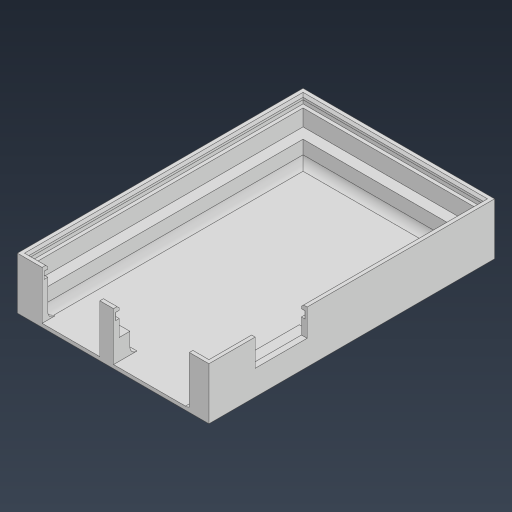
# Autodesk Inventor part: case
Saved by Autodesk Inventor 2023 (Build 270158000, 158)
## iProperties
Created: 2025-06-15
Part Number: case
Material: Generic
Document SubType Name: Modeling
Designer: szymo
Density: 1 g/cm^3
Appearance: Default
Author: szymo
Autodesk Inventor part; units mm, degrees
ref_plane "YZ Plane" through (0, 0, 0) normal (1, 0, 0) x (0, 1, 0)
ref_plane "Work Plane1" through (-26.0554, 5.5841, 57.3172) normal (0, -1, 0) x (1, 0, 0)
sketch "Sketch1" plane through (-26.0554, 5.5841, 57.3172) normal (0, -1, 0) x (1, 0, 0)
  arc A0 (-6.2529, -16.6318) -> (-5.7152, -17.8896) centre (-4.5084, -16.63) ccw projected
  line L0 (-6.2529, -16.6318) -> (-8.9554, -15.4715) projected
  arc A1 (-8.9554, -15.4715) -> (-9.6085, -15.4715) centre (-9.2819, -16.2321) ccw projected
  line L1 (-9.6085, -15.4715) -> (-11.5974, -15.1528) projected
  arc A2 (-11.5974, -15.1528) -> (-12.113, -13.8772) centre (-12.9119, -14.9421) ccw projected
  line L2 (-12.113, -13.8772) -> (-12.113, -11.7599) projected
  line L3 (-12.113, -11.7599) -> (-10.8096, -8.0503) projected
  line L4 (-10.8096, -8.0503) -> (-0.9192, -8.5103) projected
  arc A3 (-0.3314, -8.8426) -> (-0.9192, -8.5103) centre (-0.954, -9.258) ccw projected
  line L5 (-0.3314, -8.8426) -> (2.5309, -17.8896) projected
  arc A4 (2.5309, -18.6308) -> (2.5309, -17.8896) centre (1.3597, -18.2602) ccw projected
  line L6 (2.5309, -18.6308) -> (1.3597, -25.9399) projected
  line L7 (1.3597, -25.9399) -> (-2.6315, -30.1057) projected
  arc A5 (-3.5771, -30.3612) -> (-2.6315, -30.1057) centre (-3.3161, -29.4497) ccw projected
  line L8 (-3.5771, -30.3612) -> (-8.4584, -28.2656) projected
  arc A6 (-9.8385, -26.6044) -> (-8.4584, -28.2656) centre (-7.5216, -26.0835) ccw projected
  line L9 (-9.8385, -26.6044) -> (-9.8385, -22.4387) projected
  arc A7 (-9.6085, -21.9531) -> (-9.8385, -22.4387) centre (-9.2109, -22.4387) ccw projected
  line L10 (-9.6085, -21.9531) -> (-5.7152, -17.8896) projected
  line L11 (7.08, -38.1436) -> (-17.82, -38.1436) projected
  line L12 (7.08, 0) -> (7.08, -38.1436) projected
  line L13 (-17.12, 0) -> (7.08, 0) projected
  line L14 (-17.82, -38.1436) -> (-17.12, 0) projected
  line L15 (-15.12, 0) -> (-15.12, -2.1) projected
  line L16 (4.83, 0) -> (4.83, -2.3) projected
  line L17 (-7.5, -2.1) -> (-7.5, 0) projected
  line L18 (-5.08, 0) -> (-5.08, -2.1) projected
  line L19 (8.08, -39.1436) -> (-18.8385, -39.1436)
  line L20 (-18.8385, -39.1436) -> (-18.1018, 1)
  line L21 (-18.1018, 1) -> (8.08, 1)
  line L22 (8.08, 1) -> (8.08, -39.1436)
  line L23 (-18.8385, -39.1436) -> (-18.8385, 1)
  line L24 (-18.8385, 1) -> (-18.1018, 1)
  point P0 (26.0554, -57.3172)
  dimension "d2" = 1
  constraints: 12 end point, 1 parallel, 1 perpendicular, 3 other
  measures "d2" distance between parallel lines of L12 L22
extrude "Extrusion1" add sketch "Sketch1" along normal blind 0.5 contours L0 A1 L1 A2 L2 L3 L4 A3 L5 A4 L6 L7 A5 L8 A6 L9 A7 L10 A0 | L11 L14 L13 L12 | L19 L20 L21 L22 | L23 L24 L20
sketch "Sketch2" plane through (-26.0554, 5.5841, 57.3172) normal (0, 1, 0) x (1, 0, 0)
  line L0 (5.08, 0) -> (5.08, 2.1)
  line L1 (5.08, 2.1) -> (5.08, 0)
  line L2 (-5.08, 0) -> (-5.08, 2.1)
  line L3 (-7.5, 2.1) -> (-7.5, 0)
  line L4 (-15.12, 0) -> (-15.12, 2.1)
  line L5 (4.83, 2.3) -> (2.79, 2.3)
  line L6 (8.08, 39.1436) -> (8.08, -1)
  line L7 (-18.8385, 39.1436) -> (8.08, 39.1436)
  line L8 (5.08, 2.1) -> (5.08, 2.3)
  line L9 (5.08, 2.3) -> (4.83, 2.3)
  line L10 (2.79, 2.3) -> (-5.08, 2.3)
  line L11 (-5.08, 2.3) -> (-5.08, 2.0628)
  line L12 (-7.5, 2.1) -> (-7.5, 2.3)
  line L13 (-7.5, 2.3) -> (-15.12, 2.3)
  line L14 (-15.12, 2.3) -> (-15.12, 2.0628)
  line L15 (-7.5, 0) -> (-15.12, 0)
  line L16 (-5.08, 0) -> (5.08, 0)
  line L17 (8.08, -1) -> (-17.1109, -1)
  line L18 (-7.25, 2.55) -> (-15.37, 2.55)
  line L19 (-15.37, 2.55) -> (-15.37, -1)
  line L20 (-15.37, -1) -> (-7.25, -1)
  line L21 (-7.25, -1) -> (-7.25, 2.55)
  line L22 (-5.33, -1) -> (5.33, -1)
  line L23 (5.33, -1) -> (5.33, 2.55)
  line L24 (5.33, 2.55) -> (-5.33, 2.55)
  line L25 (-5.33, 2.55) -> (-5.33, -1)
  line L26 (8.08, -1) -> (-18.8385, -1)
  line L27 (-18.8385, -1) -> (-18.8385, 39.1436)
  line L28 (7.28, -0.2) -> (7.28, 38.3436)
  line L29 (7.28, 38.3436) -> (-18.0385, 38.3436)
  line L30 (-18.0385, 38.3436) -> (-18.0385, -0.2)
  line L31 (-18.0385, -0.2) -> (7.28, -0.2)
  point P0 (26.0554, 57.3172)
  point P1 (-5.33, -0.2)
  point P2 (-7.25, -0.2)
  point P3 (-7.25, -1)
  point P4 (-17.6109, -0.5)
  point P5 (-15.37, -0.2)
  point P6 (5.33, -0.2)
  point P7 (5.33, -1)
  point P8 (-17.1109, -1)
extrude "Extrusion2" add sketch "Sketch2" along normal blind 5.2 contours L6 L17 L23 L31 L28 L29 L30 L19 L26 L27 L7 | L17 L21 L31 L25
sketch "Sketch3" plane through (-17.9754, 5.0841, 58.3172) normal (1, 0, 0) x (0, 0, -1)
  line L0 (6.5, 4) -> (13.3, 4)
  line L1 (6.5, 7.65) -> (13.8, 7.65)
  line L2 (13.8, 7.65) -> (13.8, 3.5)
  line L3 (13.8, 3.5) -> (6.5, 3.5)
  line L4 (6.5, 3.5) -> (6.5, 7.65)
  line L5 (1, 3.4) -> (39.1436, 3.4) projected
  line L6 (39.1436, 3.4) -> (39.1436, 4) projected
  line L7 (13.3, 4) -> (39.1436, 4) projected
  line L8 (13.3, 4) -> (13.3, 7.15) projected
  line L9 (7, 7.15) -> (13.3, 7.15) projected
  line L10 (7, 4) -> (7, 7.15) projected
  line L11 (1, 4) -> (7, 4) projected
  line L12 (1, 3.4) -> (1, 4) projected
  point P0 (58.3172, -5.0841)
  dimension "d14" = 0.5
  dimension "d41" = 0.5
  dimension "d42" = 0.5
  dimension "d43" = 0.5
  constraints: 8 end point, 2 horizontal, 1 parallel, 1 vertical, 3 other
  measures "d14" distance between parallel lines of L3 L0
  measures "d41" distance between parallel lines of L4 L10
  measures "d42" distance between parallel lines of L9 L1
extrude "Extrusion3" cut sketch "Sketch3" against normal blind 5.2 contours L4 L1 L2 L7 L8 L9 L10 L0 | L0 L7 L2 L3 L4 | L10 L9 L8 L0
sketch "Sketch4" plane through (-26.0554, 10.7841, 57.3172) normal (0, 1, 0) x (1, 0, 0)
  line L0 (8.08, 5.5) -> (7.28, 5.5) projected
  line L1 (7.28, 5.5) -> (7.28, -0.2) projected
  line L2 (7.28, -0.2) -> (5.33, -0.2) projected
  line L3 (5.33, -0.2) -> (5.33, -1) projected
  line L4 (5.33, -1) -> (8.08, -1) projected
  line L5 (8.08, -1) -> (8.08, 5.5) projected
  line L6 (7.28, 12.8) -> (8.08, 12.8) projected
  line L7 (8.08, 12.8) -> (8.08, 39.1436) projected
  line L8 (8.08, 39.1436) -> (-18.8385, 39.1436) projected
  line L9 (-18.8385, 39.1436) -> (-18.8385, -1) projected
  line L10 (-18.8385, -1) -> (-15.37, -1) projected
  line L11 (-15.37, -1) -> (-15.37, -0.2) projected
  line L12 (-15.37, -0.2) -> (-18.0385, -0.2) projected
  line L13 (-18.0385, -0.2) -> (-18.0385, 38.3436) projected
  line L14 (-18.0385, 38.3436) -> (7.28, 38.3436) projected
  line L15 (7.28, 38.3436) -> (7.28, 12.8) projected
  line L16 (-7.25, -0.2) -> (-7.25, -1) projected
  line L17 (-7.25, -1) -> (-5.33, -1) projected
  line L18 (-5.33, -1) -> (-5.33, -0.2) projected
  line L19 (-5.33, -0.2) -> (-7.25, -0.2) projected
  line L20 (-15.37, -0.2) -> (-15.37, -1) projected
  line L21 (-15.37, -0.7) -> (-18.5385, -0.7)
  line L22 (-18.5385, -0.7) -> (-18.5385, 38.8436)
  line L23 (-18.5385, 38.8436) -> (7.78, 38.8436)
  line L24 (7.78, 38.8436) -> (7.78, 12.8)
  line L25 (7.78, 5.5) -> (7.78, -0.7)
  line L26 (7.78, -0.7) -> (5.33, -0.7)
  line L27 (-7.25, -0.7) -> (-5.33, -0.7)
  point P0 (8.08, 25.9718)
  point P1 (-15.37, -0.7)
  dimension "d44" = 0.3
  dimension "d45" = 0.3
  dimension "d46" = 0.3
  dimension "d47" = 0.3
  dimension "d48" = 0.3
  dimension "d49" = 0.3
  constraints: 14 end point, 7 perpendicular, 7 point on line, 1 horizontal, 1 midpoint, 1 parallel
  measures "d44" distance between parallel lines of L17 L27
  measures "d45" distance between parallel lines of L10 L21
  measures "d46" distance between parallel lines of L9 L22
  measures "d47" distance between parallel lines of L8 L23
  measures "d48" distance from line of point (8.08, 25.972) L24
  measures "d49" distance between parallel lines of L4 L26
extrude "Extrusion4" add sketch "Sketch4" along normal blind 1 contours L5 L4 L3 L26 L25 L0 | L24 L23 L22 L21 L11 L10 L9 L8 L7 L6 | L27 L18 L17 L16
sketch "Sketch5" plane through (-26.0554, 11.7841, 57.3172) normal (0, 1, 0) x (1, 0, 0)
  line L0 (-15.37, -1) -> (-15.37, -0.2) projected
  line L1 (8.08, 12.8) -> (8.08, 39.1436) projected
  line L2 (8.08, 39.1436) -> (-18.8385, 39.1436) projected
  line L3 (-18.8385, 39.1436) -> (-18.8385, -1) projected
  line L4 (-18.8385, -1) -> (-15.37, -1) projected
  line L5 (7.58, 5.5) -> (7.38, 5.5) projected
  line L6 (7.38, 5.5) -> (7.38, -0.3) projected
  line L7 (7.38, -0.3) -> (5.33, -0.3) projected
  line L8 (5.33, -0.3) -> (5.33, -0.5) projected
  line L9 (5.33, -0.5) -> (7.58, -0.5) projected
  line L10 (7.58, -0.5) -> (7.58, 5.5) projected
  line L11 (-7.25, -0.2) -> (-7.25, -1) projected
  line L12 (-7.25, -1) -> (-5.33, -1) projected
  line L13 (-15.37, -1) -> (-15.37, -0.2) projected
  line L14 (-15.37, -0.2) -> (-18.0385, -0.2) projected
  line L15 (-18.0385, -0.2) -> (-18.0385, 38.3436) projected
  line L16 (-18.0385, 38.3436) -> (7.28, 38.3436) projected
  line L17 (7.28, 38.3436) -> (7.28, 12.8) projected
  line L18 (-5.33, -0.2) -> (-7.25, -0.2) projected
  line L19 (-7.25, -0.2) -> (-7.25, -1) projected
  line L20 (7.28, 5.5) -> (7.28, -0.2) projected
  line L21 (7.28, -0.2) -> (5.33, -0.2) projected
  line L22 (-7.25, -0.2) -> (-7.25, -1) projected
  line L23 (-15.37, -1) -> (-15.37, -0.2) projected
  line L24 (-15.37, -0.2) -> (-18.0385, -0.2) projected
  line L25 (-18.0385, -0.2) -> (-18.0385, 38.3436) projected
  line L26 (-18.0385, 38.3436) -> (7.28, 38.3436) projected
  line L27 (-15.37, -1) -> (-15.37, -0.2) projected
  line L28 (-15.37, -0.2) -> (-18.0385, -0.2) projected
  line L29 (-18.0385, -0.2) -> (-18.0385, 38.3436) projected
  line L30 (-18.0385, 38.3436) -> (7.28, 38.3436) projected
  line L31 (7.28, 38.3436) -> (7.28, 12.8) projected
  line L32 (-7.25, -0.2) -> (-7.25, -1) projected
  line L33 (7.28, -0.2) -> (5.33, -0.2) projected
  line L34 (7.28, 12.8) -> (8.08, 12.8) projected
  line L35 (8.08, 12.8) -> (8.08, 39.1436) projected
  line L36 (8.08, 39.1436) -> (-18.8385, 39.1436) projected
  line L37 (-18.8385, 39.1436) -> (-18.8385, -1) projected
  line L38 (-18.8385, -1) -> (-15.37, -1) projected
  line L39 (8.08, -1) -> (8.08, 5.5) projected
  line L40 (8.08, 5.5) -> (7.28, 5.5) projected
  line L41 (7.28, 38.3436) -> (7.28, 12.8) projected
  line L42 (7.28, 12.8) -> (8.08, 12.8) projected
  line L43 (8.08, 12.8) -> (8.08, 39.1436) projected
  line L44 (8.08, 39.1436) -> (-18.8385, 39.1436) projected
  line L45 (-18.8385, 39.1436) -> (-18.8385, -1) projected
  line L46 (-18.8385, -1) -> (-15.37, -1) projected
  line L47 (8.08, -1) -> (8.08, 5.5) projected
  line L48 (8.08, 5.5) -> (7.28, 5.5) projected
  line L49 (7.28, 5.5) -> (7.28, -0.2) projected
  line L50 (7.28, 12.8) -> (8.08, 12.8) projected
  line L51 (8.08, 12.8) -> (8.08, 39.1436) projected
  line L52 (8.08, 39.1436) -> (-18.8385, 39.1436) projected
  line L53 (-18.8385, 39.1436) -> (-18.8385, -1) projected
  line L54 (-18.8385, -1) -> (-15.37, -1) projected
  line L55 (8.08, -1) -> (8.08, 5.5) projected
  line L56 (8.08, 5.5) -> (7.28, 5.5) projected
  line L57 (7.28, 5.5) -> (7.28, -0.2) projected
  line L58 (8.08, -1) -> (8.08, 5.5) projected
  line L59 (8.08, 5.5) -> (7.28, 5.5) projected
  line L60 (7.28, 5.5) -> (7.28, -0.2) projected
  line L61 (-5.33, -0.2) -> (-7.25, -0.2) projected
  line L62 (-7.25, -1) -> (-5.33, -1) projected
  line L63 (-5.33, -1) -> (-5.33, -0.2) projected
  line L64 (-5.33, -0.2) -> (-7.25, -0.2) projected
  line L65 (5.33, -0.2) -> (5.33, -1) projected
  line L66 (5.33, -1) -> (8.08, -1) projected
  line L67 (-7.25, -1) -> (-5.33, -1) projected
  line L68 (-5.33, -1) -> (-5.33, -0.2) projected
  line L69 (7.28, -0.2) -> (5.33, -0.2) projected
  line L70 (5.33, -0.2) -> (5.33, -1) projected
  line L71 (5.33, -1) -> (8.08, -1) projected
  line L72 (-7.25, -1) -> (-5.33, -1) projected
  line L73 (-5.33, -1) -> (-5.33, -0.2) projected
  line L74 (-5.33, -0.2) -> (-7.25, -0.2) projected
  line L75 (5.33, -0.2) -> (5.33, -1) projected
  line L76 (5.33, -1) -> (8.08, -1) projected
  line L77 (-5.33, -1) -> (-5.33, -0.2) projected
  line L78 (7.28, -0.2) -> (5.33, -0.2) projected
  line L79 (5.33, -0.2) -> (5.33, -1) projected
  line L80 (5.33, -1) -> (8.08, -1) projected
  line L81 (-15.37, -0.2) -> (-18.0385, -0.2) projected
  line L82 (-18.0385, -0.2) -> (-18.0385, 38.3436) projected
  line L83 (-18.0385, 38.3436) -> (7.28, 38.3436) projected
  line L84 (7.28, 38.3436) -> (7.28, 12.8) projected
  line L85 (7.28, 12.8) -> (8.08, 12.8) projected
  point P0 (26.0554, 57.3172)
extrude "Extrusion5" add sketch "Sketch5" along normal blind 0.6
chamfer "Chamfer1" distance 0.3 angle 45 7 edges at (-42.7597, 12.3841, 57.5172) (-44.0939, 12.3841, 38.2454) (-31.4347, 12.3841, 18.9736) (-18.7754, 12.3841, 31.7454) (-32.3454, 12.3841, 57.5172) (-18.7754, 12.3841, 54.6672) (-19.7504, 12.3841, 57.5172)
ref_plane "Work Plane2" through (-31.4254, 8.4841, 38.2454) normal (0, -1, 0) x (1, 0, 0)
sketch "Sketch6" plane through (-31.4254, 8.4841, 38.2454) normal (0, -1, 0) x (1, 0, 0)
  line L0 (-10, 19.2718) -> (-10, 20.0718) projected
  line L1 (-1.88, 20.0718) -> (-10, 20.0718) projected
  line L2 (-1.88, 20.0718) -> (-1.88, 19.2718) projected
  line L3 (-1.88, 19.2718) -> (0.04, 19.2718) projected
  line L4 (0.04, 19.2718) -> (0.04, 20.0718) projected
  line L5 (10.7, 20.0718) -> (0.04, 20.0718) projected
  line L6 (10.7, 20.0718) -> (10.7, 19.2718) projected
  line L7 (10.7, 19.2718) -> (12.65, 19.2718) projected
  line L8 (12.65, 19.2718) -> (12.65, -19.2718) projected
  line L9 (12.65, -19.2718) -> (-12.6685, -19.2718) projected
  line L10 (-12.6685, -19.2718) -> (-12.6685, 19.2718) projected
  line L11 (-12.6685, 19.2718) -> (-10, 19.2718) projected
  line L12 (-11.1685, -17.7718) -> (11.15, -17.7718)
  line L13 (11.15, -17.7718) -> (11.15, 17.7718)
  line L14 (11.15, 17.7718) -> (9.2, 17.7718)
  line L15 (9.2, 17.7718) -> (9.2, 18.5718)
  line L16 (9.2, 18.5718) -> (1.54, 18.5718)
  line L17 (1.54, 18.5718) -> (1.54, 17.7718)
  line L18 (1.54, 17.7718) -> (-3.38, 17.7718)
  line L19 (-3.38, 17.7718) -> (-3.38, 18.5718)
  line L20 (-3.38, 18.5718) -> (-8.5, 18.5718)
  line L21 (-8.5, 18.5718) -> (-8.5, 17.7718)
  line L22 (-8.5, 17.7718) -> (-11.1685, 17.7718)
  line L23 (-11.1685, 17.7718) -> (-11.1685, -17.7718)
  line L24 (-11.1685, 17.7718) -> (-11.1685, 19.2718)
  line L25 (11.15, 17.7718) -> (11.15, 19.2718)
  line L26 (-1.88, 19.2718) -> (-1.88, 17.7718)
  line L27 (0.04, 19.2718) -> (0.04, 17.7718)
  line L28 (11.15, -2.0718) -> (12.65, -2.0718)
  line L29 (12.65, -19.2718) -> (12.65, 6.2718) projected
  line L30 (11.15, 5.0718) -> (12.65, 5.0718)
  point P0 (31.4254, -38.2454)
  point P1 (12.45, 19.0718)
  point P2 (12.45, -19.0718)
  point P3 (12.65, 5.0718)
  point P4 (12.65, -2.0718)
  dimension "d50" = 1.5
  dimension "d51" = 17
  dimension "d52" = 14
  constraints: 36 end point, 8 point on line, 6 perpendicular, 13 other
  measures "d50" distance between parallel lines of L9 L12
  measures "d51" distance from line of L28 point (12.45, -19.072)
  measures "d52" distance from line of point (12.45, 19.072) L30
extrude "Extrusion6" add sketch "Sketch6" along normal up to surface (2.9 mm away) contours L24 L23 L12 L13 L28 L8 L9 L10 L11 | L3 L27 L18 L26 | L30 L13 L25 L7 L8
fillet "Fillet2" radius 1 7 edges at (-42.5939, 5.5841, 38.9954) (-42.0097, 5.5841, 57.5172) (-32.3454, 5.5841, 56.0172) (-20.2754, 5.5841, 50.4172) (-18.7754, 5.5841, 39.7454) (-20.2754, 5.5841, 28.3236) (-31.4347, 5.5841, 20.4736)
equation "\"d45\" = d44"
equation "\"d46\" = d44"
equation "\"d47\" = d44"
equation "\"d48\" = d44"
equation "\"d49\" = d44"
body "Solid1"
